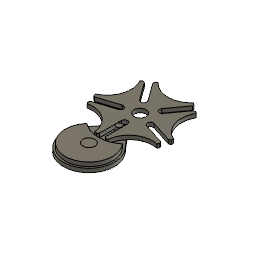
geneva wheel mechanism (Autodesk Fusion 360 design; units mm, degrees)
part number: 2026-03-23-16-24-24-879
part number: 2026-03-23-16-39-09-306
part number: 2026-03-23-16-44-08-491
part number: 2026-03-23-16-54-27-971
part number: 2026-03-23-16-55-45-334
Autodesk Fusion 360 part; units mm, degrees
note: some values were not read from the file. Set by a fixed rule: which sketch regions a step uses.
sketch "Sketch1" plane through (0, 0, 0) normal (0, 1, 0) x (1, 0, 0) in component "follower"
  line L0 (0, 0) -> (29.3893, -40.4508) construction
  line L1 (0, 0) -> (50, 0) construction
  line L2 (0, 0) -> (-29.3893, -40.4508) construction
  line L3 (0, 0) -> (50, 0) construction
  line L4 (8.7219, -18.3845) -> (26.3554, -42.655)
  line L5 (32.4231, -38.2467) -> (14.7895, -13.9761)
  arc A0 (14.7895, -13.9761) -> (8.7219, -18.3845) centre (11.7557, -16.1803) ccw
  line L6 (11.7557, -16.1803) -> (29.3893, -40.4508) construction
  line L7 (20.1799, 2.6139) -> (48.7116, 11.8844)
  arc A1 (17.8623, 9.7468) -> (20.1799, 2.6139) centre (19.0211, 6.1803) ccw
  line L8 (46.394, 19.0173) -> (17.8623, 9.7468)
  line L9 (3.75, 20) -> (3.75, 50)
  arc A2 (-3.75, 20) -> (3.75, 20) centre (0, 20) ccw
  line L10 (-3.75, 50) -> (-3.75, 20)
  line L11 (-17.8623, 9.7468) -> (-46.394, 19.0173)
  arc A3 (-20.1799, 2.6139) -> (-17.8623, 9.7468) centre (-19.0211, 6.1803) ccw
  line L12 (-48.7116, 11.8844) -> (-20.1799, 2.6139)
  line L13 (-14.7895, -13.9761) -> (-32.4231, -38.2467)
  arc A4 (-8.7219, -18.3845) -> (-14.7895, -13.9761) centre (-11.7557, -16.1803) ccw
  line L14 (-26.3554, -42.655) -> (-8.7219, -18.3845)
  circle A5 centre (0, 0) radius 7.5
  arc A6 (-31.5791, -43.4951) -> (-18.1729, -31.3928) centre (0, -65) ccw construction
  arc A7 (22.1872, -44.8077) -> (-22.1872, -44.8077) centre (0, -65) ccw
  arc A8 (-26.2727, -42.5411) -> (-22.1872, -44.8077) centre (0, 0) ccw
  arc A9 (22.1872, -44.8077) -> (26.2727, -42.5411) centre (0, 0) ccw
  arc A10 (29.3183, -40.5023) -> (29.3893, -40.4508) centre (0, 0) ccw
  arc A11 (49.4709, 7.2549) -> (35.7584, -34.9476) centre (61.8187, -20.0861) ccw
  arc A12 (8.3875, 49.2915) -> (44.2871, 23.2089) centre (38.206, 52.5861) ccw
  arc A13 (-44.2871, 23.2089) -> (-8.3875, 49.2915) centre (-38.206, 52.5861) ccw
  arc A14 (-35.7584, -34.9476) -> (-49.4709, 7.2549) centre (-61.8187, -20.0861) ccw
  arc A15 (-48.5777, 11.8409) -> (-49.4709, 7.2549) centre (0, 0) ccw
  arc A16 (-35.7584, -34.9476) -> (-32.3403, -38.1327) centre (0, 0) ccw
  arc A17 (32.3403, -38.1327) -> (35.7584, -34.9476) centre (0, 0) ccw
  arc A18 (49.4709, 7.2549) -> (48.5777, 11.8409) centre (0, 0) ccw
  arc A19 (46.2601, 18.9738) -> (44.2871, 23.2089) centre (0, 0) ccw
  arc A20 (8.3875, 49.2915) -> (3.75, 49.8592) centre (0, 0) ccw
  arc A21 (-3.75, 49.8592) -> (-8.3875, 49.2915) centre (0, 0) ccw
  arc A22 (-44.2871, 23.2089) -> (-46.2601, 18.9738) centre (0, 0) ccw
  dimension "d1" = 100
  dimension "d2" = 50
  dimension "d3" = 54
  dimension "d4" = 126
  dimension "d5" = 65
  dimension "d6" = 60
  dimension "d8" = 20
  dimension "d11" = 15
  dimension "d13" = 360
  constraint coincident L0.start L1.start
  constraint horizontal L1
  constraint horizontal L3
  constraint tangent L0 A6
  constraint tangent L2 A6
  constraint concentric A6 A7
  constraint parallel L4 L5
  constraint tangent L5 A0
  constraint tangent L4 A0
  constraint coincident L0.end L6.end
  constraint parallel L0 L6
  constraint coincident L13 A16.end
  constraint coincident L14 A6.end
  constraint coincident L14 A8.start
  constraint concentric A8 A16
  constraint coincident L5 A17.start
  constraint concentric A10 A17
  constraint coincident L4 A9.end
  constraint coincident A6 A10.start
  constraint concentric A9 A10
  constraint coincident L7 A18.end
  constraint coincident L8 A19.start
  constraint concentric A18 A19
  constraint coincident L9 A20.end
  constraint coincident L10 A21.start
  constraint concentric A20 A21
  constraint coincident L11 A22.end
  constraint coincident L12 A15.start
  constraint concentric A15 A22
  constraint concentric A15 A16
  constraint concentric A17 A18
  constraint concentric A19 A20
  constraint concentric A21 A22
  measures "d1" diameter of A8
  measures "d2" distance of L0.start L0.end
  measures "d3" angle of L0 L1
  measures "d4" angle of L2 L3
  measures "d5" distance of L0.start A6.centre
  measures "d6" diameter of A7
  measures "d8" distance of L0.start A0.centre
  measures "d11" diameter of A5
extrude "Extrude1" add sketch "Sketch1" along normal blind 5 makes body 1 in component "follower"
chamfer "Chamfer1" distance 2 angle 45 10 edges at (26.2727, 2.5, 42.5411) (32.3403, 2.5, 38.1327) (48.5777, 2.5, -11.8409) (46.2601, 2.5, -18.9738) (3.75, 2.5, -49.8592) (-3.75, 2.5, -49.8592) (-46.2601, 2.5, -18.9738) (-48.5777, 2.5, -11.8409) (-32.3403, 2.5, 38.1327) (-26.2727, 2.5, 42.5411) on bodies 1 in component "follower"
sketch "Sketch1 (2)" plane through (0, 5, 0) normal (0, 1, 0) x (-1, 0, 0) in component "cam"
  line L0 (25.0971, 40.9231) -> (24.5504, 43.5578)
  arc A0 (24.5504, 43.5578) -> (22.1872, 44.8077) centre (0, 0) ccw
  arc A1 (-22.1872, 44.8077) -> (22.1872, 44.8077) centre (0, 65) ccw
  arc A2 (-22.1872, 44.8077) -> (-24.5504, 43.5578) centre (0, 0) ccw
  line L1 (-24.5504, 43.5578) -> (-25.0971, 40.9231)
  line L2 (-25.0971, 40.9231) -> (-8.7219, 18.3845)
  arc A3 (-14.7895, 13.9761) -> (-8.7219, 18.3845) centre (-11.7557, 16.1803) ccw
  line L3 (-14.7895, 13.9761) -> (-31.1647, 36.5147)
  line L4 (-31.1647, 36.5147) -> (-33.8394, 36.8089)
  arc A4 (-33.8394, 36.8089) -> (-35.7584, 34.9476) centre (0, 0) ccw
  arc A5 (-49.4709, -7.2549) -> (-35.7584, 34.9476) centre (-61.8187, 20.0861) ccw
  arc A6 (-49.4709, -7.2549) -> (-49.0124, -9.8887) centre (0, 0) ccw
  line L5 (-49.0124, -9.8887) -> (-46.6756, -11.2228)
  line L6 (-46.6756, -11.2228) -> (-20.1799, -2.6139)
  arc A7 (-17.8623, -9.7468) -> (-20.1799, -2.6139) centre (-19.0211, -6.1803) ccw
  line L7 (-17.8623, -9.7468) -> (-44.358, -18.3558)
  line L8 (-44.358, -18.3558) -> (-45.4643, -20.8086)
  arc A8 (-45.4643, -20.8086) -> (-44.2871, -23.2089) centre (0, 0) ccw
  arc A9 (-8.3875, -49.2915) -> (-44.2871, -23.2089) centre (-38.206, -52.5861) ccw
  arc A10 (-8.3875, -49.2915) -> (-5.741, -49.6693) centre (0, 0) ccw
  line L9 (-5.741, -49.6693) -> (-3.75, -47.8592)
  line L10 (-3.75, -47.8592) -> (-3.75, -20)
  arc A11 (3.75, -20) -> (-3.75, -20) centre (0, -20) ccw
  line L11 (3.75, -20) -> (3.75, -47.8592)
  line L12 (3.75, -47.8592) -> (5.741, -49.6693)
  arc A12 (5.741, -49.6693) -> (8.3875, -49.2915) centre (0, 0) ccw
  arc A13 (44.2871, -23.2089) -> (8.3875, -49.2915) centre (38.206, -52.5861) ccw
  arc A14 (44.2871, -23.2089) -> (45.4643, -20.8086) centre (0, 0) ccw
  line L13 (45.4643, -20.8086) -> (44.358, -18.3558)
  line L14 (44.358, -18.3558) -> (17.8623, -9.7468)
  arc A15 (20.1799, -2.6139) -> (17.8623, -9.7468) centre (19.0211, -6.1803) ccw
  line L15 (20.1799, -2.6139) -> (46.6756, -11.2228)
  line L16 (46.6756, -11.2228) -> (49.0124, -9.8887)
  arc A16 (49.0124, -9.8887) -> (49.4709, -7.2549) centre (0, 0) ccw
  arc A17 (35.7584, 34.9476) -> (49.4709, -7.2549) centre (61.8187, 20.0861) ccw
  arc A18 (35.7584, 34.9476) -> (33.8394, 36.8089) centre (0, 0) ccw
  line L17 (33.8394, 36.8089) -> (31.1647, 36.5147)
  line L18 (31.1647, 36.5147) -> (14.7895, 13.9761)
  arc A19 (8.7219, 18.3845) -> (14.7895, 13.9761) centre (11.7557, 16.1803) ccw
  line L19 (8.7219, 18.3845) -> (25.0971, 40.9231)
  circle A20 centre (0, 0) radius 7.5
  arc A21 (31.5791, 43.4951) -> (18.1729, 31.3928) centre (0, 65) ccw
  circle A22 centre (0, 65) radius 30
  circle A23 centre (0, 65) radius 32.5
  circle A24 centre (0, 65) radius 7.5
  line L20 (0, 0) -> (0, 35)
  circle A25 centre (0, 26.794) radius 3.75
  line L21 (24.6979, 43.875) -> (3.7997, 19.4423)
  line L22 (-3.7997, 19.4423) -> (-24.6979, 43.875)
  arc A26 (-3.7997, 19.4423) -> (3.7997, 19.4423) centre (0, 22.6923) ccw
  arc A27 (22.3607, 45) -> (-22.3607, 45) centre (0, 18.0742) ccw
  point P0 (0, 15)
  dimension "d17" = 60
  dimension "d18" = 65
  dimension "d19" = 15
  dimension "d20" = 7.5
  dimension "d21" = 15
  dimension "d22" = 5
  dimension "d23" = 20
  dimension "d24" = 35
  constraint concentric A1 A22
  constraint concentric A21 A23
  constraint concentric A1 A24
  constraint coincident A0.centre A2.centre
  constraint midpoint A1 L20.end
  constraint coincident A21 A25.centre
  constraint coincident L20 A25.centre
  constraint coincident A23 L21.start
  constraint coincident L20 P0
  constraint coincident A23 L22.end
  constraint tangent A23 L21
  constraint tangent A23 L22
  constraint coincident P0 L21
  constraint coincident P0 L22
  constraint tangent L21 A26
  constraint tangent L22 A26
  constraint coincident A22 A27.end
  constraint coincident A22 A27.start
  constraint horizontal A27.start A27.end
  measures "d17" diameter of A22
  measures "d18" diameter of A23
  measures "d19" diameter of A24
  measures "d20" diameter of A25
  measures "d21" distance of P0 A0.centre
  measures "d22" radius of A26
  measures "d23" vertical distance of A1.centre A27.start
  measures "d24" radius of A27
extrude "Extrude1'" add sketch "Sketch1 (2)" against normal blind 5 separate body contours A0 A1 A22 A23 L20 | A21 A23 L20 A25 L21 | A0 A2 A22 A23 L21 L22 | A21 L20 A25 L21 A26 | A1 A22 A27 | A21 A23 L20 A25 L22 | A1 A2 A22 A23 L20 | A21 L20 A25 | A21 L20 A25 | A22 A27 | A21 L20 A25 | A21 L20 A25 | A21 L20 A25 L22 A26 makes body 2 in component "cam"
extrude "Extrude2" add sketch "Sketch1 (2)" along normal blind 5 contours A21 L20 A25 | A21 L20 A25 | A22 A27 | A21 L20 A25 | A21 L20 A25 bodies 2 in component "cam"
cylinder "CylinderPrimitive1" add diameter 15 height -20 placed x (1, 0, 0) y (0, 0, -1) z (0, 1, 0) at (0, 5, 0) separate body makes body 3 in component "shaft"
sketch "Sketch1 (3)" plane through (0, 0, 0) normal (0, 1, 0) x (1, 0, 0) in component "Component"
  circle A0 centre (0, -65) radius 7.5
  circle A1 centre (0, -65) radius 7.5
  arc A2 (-22.3607, -45) -> (22.3607, -45) centre (0, -65) ccw
  arc A3 (-22.3607, -45) -> (22.3607, -45) centre (0, -18.0742) ccw
  dimension "d33" = 15
  constraint coincident A0.centre A1.centre
  measures "d33" diameter of A0
extrude "Extrude1''" add sketch "Sketch1 (3)" along normal blind -15 and the other way blind -5 separate body contours A0 A1 makes body 4 in component "Component"
component "cam" placed x (1, 0, 0) y (0, 1, 0) z (0, 0, 1) at (0, -5, 0)
component "shaft" placed x (1, 0, 0) y (0, 1, 0) z (0, 0, 1) at (0, 0, 0)
component "follower" placed x (0.809017, 0, -0.587785) y (0, 1, 0) z (0.587785, 0, 0.809017) at (0, 0, 0)
component "Component" placed x (1, 0, 0) y (0, 1, 0) z (0, 0, 1) at (0, 0, 0)
equation "d4 = 180 deg - 54 deg"
